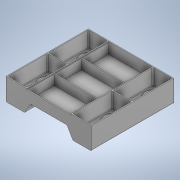
# Autodesk Inventor part: WarSunTray
Saved by Autodesk Inventor 2021 (Build 250183000, 183)
## iProperties
Created: 2023-03-17
Part Number: WarSunTray
Material: ABS Plastic
Document SubType Name: Modeling
Designer: Bradley
Density: 1.06 g/cm^3
Appearance: Smooth - Medium Gray
Author: Bradley
Autodesk Inventor part; units mm, degrees
ref_plane "YZ Plane" through (0, 0, 0) normal (1, 0, 0) x (0, 1, 0)
ref_plane "XZ Plane" through (0, 0, 0) normal (0, 1, 0) x (-1, 0, 0)
ref_plane "XY Plane" through (0, 0, 0) normal (0, 0, 1) x (1, 0, 0)
sketch "Sketch1" plane through (0, 0, 0) normal (0, 0, 1) x (1, 0, 0)
  line L0 (-74, 20.1) -> (-74, -17.9)
  line L1 (-74, -17.9) -> (-41.627, -17.9)
  line L2 (-41.627, -17.9) -> (-31.2924, 0)
  line L3 (-31.2924, 0) -> (31.2924, 0)
  line L4 (31.2924, 0) -> (41.627, -17.9)
  line L5 (41.627, -17.9) -> (74, -17.9)
  line L6 (74, -17.9) -> (74, 20.1)
  line L7 (-74, 20.1) -> (74, 20.1)
  line L8 (-31.2924, -0.5) -> (31.2924, -0.5) construction
  line L9 (31.2924, -0.5) -> (62.5848, -54.7) construction
  line L10 (62.5848, -54.7) -> (31.2924, -108.9) construction
  line L11 (31.2924, -108.9) -> (-31.2924, -108.9) construction
  line L12 (-31.2924, -108.9) -> (-62.5848, -54.7) construction
  line L13 (-62.5848, -54.7) -> (-31.2924, -0.5) construction
  point P0 (0, 0)
  point P1 (0, 0)
  point P2 (0, 20.1)
  point P3 (0, -54.7)
  dimension "d0" = 74
  dimension "d2" = 38
  dimension "d3" = 108.4
  dimension "d4" = 0.5
  dimension "d5" = 0.25
  dimension "d6" = 91
  dimension "d53" = 20.1
  constraints: 28 end point, 2 horizontal, 2 midpoint, 2 parallel, 2 perpendicular, 2 point on line, 2 vertical alignment, 1 coincident, 1 collinear, 1 vertical, 13 other
  measures "d0" distance from line of point (0, 0) L0
  measures "d2" distance of L0.start L0.end
  measures "d3" distance between parallel lines of L11 L8
  measures "d4" distance between parallel lines of L8 L3
  measures "d5" distance between parallel lines of L13 L2
  measures "d6" distance between parallel lines of L11 L1
  measures "d53" distance between parallel lines of L3 L7
extrude "Extrusion1" add sketch "Sketch1" along normal mid plane 142.25
fillet "Fillet1" radius 2 6 edges at (-31.2924, 0, 0) (31.2924, 0, 0) (41.627, -17.9, 0) (-41.627, -17.9, 0) (-74, -17.9, 0) (74, -17.9, 0)
sketch "Sketch2" plane through (-74, 20.1, 71.125) normal (0, 1, 0) x (1, 0, 0)
  line L0 (0, 142.25) -> (0, 0) projected
  line L1 (148, 0) -> (0, 0) projected
  line L2 (148, 142.25) -> (148, 0) projected
  line L3 (0, 142.25) -> (148, 142.25) projected
  circle A0 centre (18.1, 124.15) radius 16 construction
  circle A1 centre (18.1, 124.15) radius 16.5 construction
  circle A2 centre (18.1, 124.15) radius 11.5 construction
  circle A3 centre (18.1, 124.15) radius 12
  circle A4 centre (18.1, 124.15) radius 18.1 construction
  line L4 (0, 142.25) -> (148, 142.25) construction
  circle A5 centre (129.9, 18.1) radius 18.1 construction
  line L5 (148, 142.25) -> (148, 0) construction
  line L6 (148, 0) -> (0, 0) construction
  line L7 (0, 142.25) -> (0, 0) construction
  line L8 (18.1, 124.15) -> (18.1, 140.65) construction
  line L9 (3.6, 140.65) -> (32.6, 140.65)
  line L10 (34.6, 138.65) -> (34.6, 73.925)
  line L11 (32.6, 71.925) -> (3.6, 71.925)
  line L12 (1.6, 73.925) -> (1.6, 138.65)
  arc A6 (3.6, 140.65) -> (1.6, 138.65) centre (3.6, 138.65) ccw
  arc A7 (34.6, 138.65) -> (32.6, 140.65) centre (32.6, 138.65) ccw
  arc A8 (32.6, 71.925) -> (34.6, 73.925) centre (32.6, 73.925) ccw
  arc A9 (1.6, 73.925) -> (3.6, 71.925) centre (3.6, 73.925) ccw
  circle A10 centre (129.9, 124.15) radius 12
  circle A11 centre (18.1, 88.8) radius 12
  circle A12 centre (129.9, 88.8) radius 12
  circle A13 centre (18.1, 53.45) radius 12
  circle A14 centre (129.9, 53.45) radius 12
  circle A15 centre (18.1, 18.1) radius 12
  circle A16 centre (129.9, 18.1) radius 12
  arc A17 (115.4, 140.65) -> (113.4, 138.65) centre (115.4, 138.65) ccw
  line L13 (115.4, 140.65) -> (144.4, 140.65)
  line L14 (113.4, 73.925) -> (113.4, 138.65)
  arc A18 (146.4, 138.65) -> (144.4, 140.65) centre (144.4, 138.65) ccw
  line L15 (146.4, 138.65) -> (146.4, 73.925)
  line L16 (144.4, 71.925) -> (115.4, 71.925)
  arc A19 (144.4, 71.925) -> (146.4, 73.925) centre (144.4, 73.925) ccw
  arc A20 (113.4, 73.925) -> (115.4, 71.925) centre (115.4, 73.925) ccw
  arc A21 (3.6, 70.325) -> (1.6, 68.325) centre (3.6, 68.325) ccw
  line L17 (3.6, 70.325) -> (32.6, 70.325)
  line L18 (1.6, 3.6) -> (1.6, 68.325)
  arc A22 (34.6, 68.325) -> (32.6, 70.325) centre (32.6, 68.325) ccw
  line L19 (34.6, 68.325) -> (34.6, 3.6)
  line L20 (32.6, 1.6) -> (3.6, 1.6)
  arc A23 (32.6, 1.6) -> (34.6, 3.6) centre (32.6, 3.6) ccw
  arc A24 (1.6, 3.6) -> (3.6, 1.6) centre (3.6, 3.6) ccw
  arc A25 (115.4, 70.325) -> (113.4, 68.325) centre (115.4, 68.325) ccw
  line L21 (115.4, 70.325) -> (144.4, 70.325)
  line L22 (113.4, 3.6) -> (113.4, 68.325)
  arc A26 (146.4, 68.325) -> (144.4, 70.325) centre (144.4, 68.325) ccw
  line L23 (146.4, 68.325) -> (146.4, 3.6)
  line L24 (144.4, 1.6) -> (115.4, 1.6)
  arc A27 (144.4, 1.6) -> (146.4, 3.6) centre (144.4, 3.6) ccw
  arc A28 (113.4, 3.6) -> (115.4, 1.6) centre (115.4, 3.6) ccw
  circle A29 centre (129.9, 18.1) radius 16.5 construction
  point P0 (74, 71.125)
  dimension "d27" = 33
  dimension "d10" = 32
  dimension "d13" = 23
  dimension "d23" = 1.6
  dimension "d26" = 24
  dimension "d28" = 2
  dimension "d31" = 111.8
  dimension "d34" = 35.35
  dimension "d39" = 111.8
  dimension "d42" = 70.325
  dimension "d46" = 1.6
  constraints: 34 end point, 32 point on circle, 29 centre point, 14 tangent, 6 coincident, 5 vertical, 4 equal radius, 4 horizontal, 2 parallel, 1 perpendicular, 1 vertical alignment, 77 other
  measures "d10" diameter of A0
  measures "d13" diameter of A2
  measures "d26" diameter of A3
  measures "d28" radius of A6
  measures "d31" distance of A3.centre A10.centre
  measures "d34" distance of A3.centre A11.centre
  measures "d39" distance of A6.centre A17.centre
  measures "d42" distance of A6.centre A21.centre
  measures "d46" distance between parallel lines of L17 L11
extrude "Extrusion2" cut sketch "Sketch2" against normal blind 37 contours A3 | A10 | A11 | A12 | A13 | A14 | A15 | A16
extrude "Extrusion3" cut sketch "Sketch2" against normal blind 27 contours L9 A7 L10 A8 L11 A9 L12 A6 | L13 A18 L15 A19 L16 A20 L14 A17 | L17 A22 L19 A23 L20 A24 L18 A21 | L21 A26 L23 A27 L24 A28 L22 A25
chamfer "Chamfer1" distance 2 angle 45 8 edges at (-67.9, -6.9, 17.675) (-67.9, -6.9, 53.025) (-67.9, -6.9, -17.675) (-67.9, -6.9, -53.025) (43.9, -6.9, -53.025) (43.9, -6.9, -17.675) (43.9, -6.9, 17.675) (43.9, -6.9, 53.025)
fillet "Fillet2" radius 1 56 edges at (43.9, -16.9, 53.025) (43.9, -16.9, 17.675) (43.9, -16.9, -17.675) (43.9, -16.9, -53.025) (-67.9, -16.9, -53.025) (-67.9, -16.9, -17.675) (-67.9, -16.9, 53.025) (-67.9, -16.9, 17.675) (55.9, -6.9, 0.8) (39.9858, -6.9, 1.3858) (39.4, -6.9, 35.1625) (39.9858, -6.9, 68.9392) (55.9, -6.9, 69.525) (71.8142, -6.9, 68.9392) (72.4, -6.9, 35.1625) (71.8142, -6.9, 1.3858) (55.9, -6.9, -69.525) (39.9858, -6.9, -68.9392) (39.4, -6.9, -35.1625) (39.9858, -6.9, -1.3858) (55.9, -6.9, -0.8) (71.8142, -6.9, -1.3858) (72.4, -6.9, -35.1625) (71.8142, -6.9, -68.9392) (-55.9, -6.9, -0.8) (-39.9858, -6.9, -1.3858) (-39.4, -6.9, -35.1625) (-39.9858, -6.9, -68.9392) (-55.9, -6.9, -69.525) (-71.8142, -6.9, -68.9392) (-72.4, -6.9, -35.1625) (-71.8142, -6.9, -1.3858) (-55.9, -6.9, 0.8) (-71.8142, -6.9, 1.3858) (-72.4, -6.9, 35.1625) (-71.8142, -6.9, 68.9392) (-55.9, -6.9, 69.525) (-39.9858, -6.9, 68.9392) (-39.4, -6.9, 35.1625) (-39.9858, -6.9, 1.3858) (-69.9, -6.9, 17.675) (-67.9, -8.9, 17.675) (-69.9, -6.9, 53.025) (-67.9, -8.9, 53.025) (-69.9, -6.9, -17.675) (-67.9, -8.9, -17.675) (-69.9, -6.9, -53.025) (-67.9, -8.9, -53.025) (41.9, -6.9, -53.025) (43.9, -8.9, -53.025) (41.9, -6.9, -17.675) (43.9, -8.9, -17.675) (41.9, -6.9, 17.675) (43.9, -8.9, 17.675) (41.9, -6.9, 53.025) (43.9, -8.9, 53.025)
sketch "Sketch3" plane through (0, 0, 71.125) normal (0, 0, 1) x (1, 0, 0)
  arc A0 (72, -17.9) -> (74, -15.9) centre (72, -15.9) ccw projected
  line L0 (74, -15.9) -> (74, 20.1) projected
  line L1 (74, 20.1) -> (-74, 20.1) projected
  line L2 (-74, 20.1) -> (-74, -15.9) projected
  arc A1 (-74, -15.9) -> (-72, -17.9) centre (-72, -15.9) ccw projected
  line L3 (-72, -17.9) -> (-42.7817, -17.9) projected
  arc A2 (-42.7817, -17.9) -> (-41.0496, -16.9) centre (-42.7817, -15.9) ccw projected
  line L4 (-41.0496, -16.9) -> (-31.8697, -1) projected
  arc A3 (-30.1377, 0) -> (-31.8697, -1) centre (-30.1377, -2) ccw projected
  line L5 (-30.1377, 0) -> (30.1377, 0) projected
  arc A4 (31.8697, -1) -> (30.1377, 0) centre (30.1377, -2) ccw projected
  line L6 (31.8697, -1) -> (41.0496, -16.9) projected
  arc A5 (41.0496, -16.9) -> (42.7817, -17.9) centre (42.7817, -15.9) ccw projected
  line L7 (42.7817, -17.9) -> (72, -17.9) projected
  line L8 (-39.4, 20.1) -> (-39.4, -5.9) projected
  line L9 (-39.4, 20.1) -> (-39.4, -5.9) projected
  line L10 (39.4, 20.1) -> (39.4, -5.9) projected
  line L11 (39.4, 20.1) -> (39.4, -5.9) projected
  line L12 (74, 20.1) -> (-74, 20.1) projected
  line L13 (-37.8721, 20.1) -> (-38.6, 18.1)
  line L14 (-38.6, 18.1) -> (38.6, 18.1)
  line L15 (38.6, 18.1) -> (37.8721, 20.1)
  point P0 (0, 0)
  point P1 (0, 18.1)
  point P2 (0, 20.1)
  dimension "d54" = 2
  dimension "d55" = 70
  dimension "d56" = 0.7279
  dimension "d57" = 0.8
  dimension "d58" = 77.2
  constraints: 6 end point, 1 equal length, 1 horizontal, 1 midpoint, 1 vertical alignment, 4 other
  measures "d54" distance between parallel lines of L14 L1
  measures "d55" angle of L14 L13
  measures "d56" horizontal distance of L13.start L13.end
  measures "d57" distance from line of L13.end L8
  measures "d58" distance of L13.end L14.end
extrude "Extrusion4" cut sketch "Sketch3" against normal blind 140.65 contours L15 L14 L13 L1
sketch "Sketch4" plane through (-38.6, 18.1, 71.125) normal (0, 1, 0) x (1, 0, 0)
  line L0 (76.4721, 140.65) -> (76.4721, 0) projected
  line L1 (112.6, 0) -> (76.4721, 0) projected
  line L2 (112.6, 142.25) -> (112.6, 0) projected
  line L3 (-35.4, 142.25) -> (112.6, 142.25) projected
  line L4 (-35.4, 142.25) -> (-35.4, 0) projected
  line L5 (0.7279, 0) -> (-35.4, 0) projected
  line L6 (0.7279, 0) -> (0.7279, 140.65) projected
  line L7 (0.7279, 140.65) -> (76.4721, 140.65) projected
  arc A0 (80, 140.65) -> (78, 138.65) centre (80, 138.65) ccw projected
  line L8 (80, 140.65) -> (109, 140.65) projected
  arc A1 (111, 138.65) -> (109, 140.65) centre (109, 138.65) ccw projected
  line L9 (111, 138.65) -> (111, 73.925) projected
  arc A2 (109, 71.925) -> (111, 73.925) centre (109, 73.925) ccw projected
  line L10 (109, 71.925) -> (80, 71.925) projected
  arc A3 (78, 73.925) -> (80, 71.925) centre (80, 73.925) ccw projected
  line L11 (78, 73.925) -> (78, 138.65) projected
  arc A4 (-31.8, 70.325) -> (-33.8, 68.325) centre (-31.8, 68.325) ccw projected
  line L12 (-31.8, 70.325) -> (-2.8, 70.325) projected
  arc A5 (-0.8, 68.325) -> (-2.8, 70.325) centre (-2.8, 68.325) ccw projected
  line L13 (-0.8, 68.325) -> (-0.8, 3.6) projected
  arc A6 (-2.8, 1.6) -> (-0.8, 3.6) centre (-2.8, 3.6) ccw projected
  line L14 (-2.8, 1.6) -> (-31.8, 1.6) projected
  arc A7 (-33.8, 3.6) -> (-31.8, 1.6) centre (-31.8, 3.6) ccw projected
  line L15 (-33.8, 3.6) -> (-33.8, 68.325) projected
  arc A8 (80, 70.325) -> (78, 68.325) centre (80, 68.325) ccw projected
  line L16 (80, 70.325) -> (109, 70.325) projected
  arc A9 (111, 68.325) -> (109, 70.325) centre (109, 68.325) ccw projected
  line L17 (111, 68.325) -> (111, 3.6) projected
  arc A10 (109, 1.6) -> (111, 3.6) centre (109, 3.6) ccw projected
  line L18 (109, 1.6) -> (80, 1.6) projected
  arc A11 (78, 3.6) -> (80, 1.6) centre (80, 3.6) ccw projected
  line L19 (78, 3.6) -> (78, 68.325) projected
  arc A12 (-2.8, 71.925) -> (-0.8, 73.925) centre (-2.8, 73.925) ccw projected
  line L20 (-2.8, 71.925) -> (-31.8, 71.925) projected
  arc A13 (-33.8, 73.925) -> (-31.8, 71.925) centre (-31.8, 73.925) ccw projected
  line L21 (-33.8, 73.925) -> (-33.8, 138.65) projected
  arc A14 (-31.8, 140.65) -> (-33.8, 138.65) centre (-31.8, 138.65) ccw projected
  line L22 (-31.8, 140.65) -> (-2.8, 140.65) projected
  arc A15 (-0.8, 138.65) -> (-2.8, 140.65) centre (-2.8, 138.65) ccw projected
  line L23 (-0.8, 138.65) -> (-0.8, 73.925) projected
  line L24 (0.7279, 140.65) -> (76.4721, 140.65) projected
  line L25 (0.8, 140.65) -> (76.4, 140.65)
  line L26 (76.4, 140.65) -> (76.4, 1.6)
  line L27 (76.4, 1.6) -> (0.8, 1.6)
  line L28 (0.8, 1.6) -> (0.8, 140.65)
  line L29 (0.8, 95.3667) -> (76.4, 95.3667)
  line L30 (76.4, 93.7667) -> (0.8, 93.7667)
  line L31 (0.8, 48.4833) -> (76.4, 48.4833)
  line L32 (76.4, 46.8833) -> (0.8, 46.8833)
  point P0 (38.6, 71.125)
  point P1 (76.4, 71.125)
  point P2 (38.6, 1.6)
  dimension "d61" = 1.6
  dimension "d64" = 1.6
  dimension "d65" = 1.6
  dimension "d66" = 45.2833
  dimension "d67" = 45.2833
  dimension "d68" = 45.2833
  dimension "d69" = 75.6
  constraints: 16 end point, 9 point on line, 4 perpendicular, 3 parallel, 2 midpoint, 1 horizontal, 1 horizontal alignment, 1 vertical alignment
  measures "d61" distance between parallel lines of L28 L23
  measures "d64" distance between parallel lines of L30 L29
  measures "d65" distance between parallel lines of L32 L31
  measures "d66" distance between parallel lines of L25 L29
  measures "d67" distance between parallel lines of L31 L30
  measures "d68" distance between parallel lines of L27 L32
  measures "d69" distance of L30.start L30.end
extrude "Extrusion5" cut sketch "Sketch4" against normal blind 17.1 contours L26 L29 L28 L7 | L26 L31 L28 L30 | L26 L27 L28 L32
equation "\"d2\" = Depth"
equation "\"d3\" = Outside"
equation "\"d46\" = d23"
equation "\"d64\" = d61"
equation "\"d65\" = d61"
equation "\"d66\" = d68"
equation "\"d67\" = d66"
equation "\"Depth\" = 38"
equation "\"Outside\" = 108.4"
body "Solid1"
